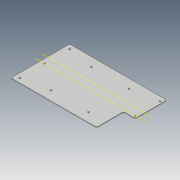
# Autodesk Inventor part: bottomMountingPlate
Saved by Autodesk Inventor 2018 (Build 220112000, 112)
## iProperties
Created: 2020-01-17
Part Number: bottomMountingPlate
Material: Generic
Document SubType Name: Modeling
Designer: anirudh.bali
Density: 1 g/cm^3
Appearance: Default
Author: anirudh.bali
Autodesk Inventor part; units mm, degrees
ref_plane "YZ Plane" through (0, 0, 0) normal (1, 0, 0) x (0, 1, 0)
ref_plane "XZ Plane" through (0, 0, 0) normal (0, 1, 0) x (-1, 0, 0)
ref_plane "XY Plane" through (0, 0, 0) normal (0, 0, 1) x (1, 0, 0)
sketch "Sketch1" plane through (0, 0, 0) normal (0, 1, 0) x (-1, 0, 0)
  line L0 (10.16, 0) -> (218.44, 0)
  line L1 (218.44, -165.1) -> (10.16, -165.1)
  circle A0 centre (218.44, -25.4) radius 1.75
  circle A1 centre (218.44, -82.55) radius 1.75
  circle A2 centre (218.44, -139.7) radius 1.75
  circle A3 centre (10.16, -25.4) radius 1.75
  circle A4 centre (10.16, -82.55) radius 1.75
  circle A5 centre (10.16, -139.7) radius 1.75
  line L2 (218.44, 0) -> (228.6, 0)
  line L3 (228.6, 0) -> (228.6, -165.1)
  line L4 (228.6, -165.1) -> (218.44, -165.1)
  line L5 (10.16, 0) -> (0, 0)
  line L6 (0, 0) -> (0, -165.1)
  line L7 (0, -165.1) -> (10.16, -165.1)
  dimension "d18" = 3.5
  dimension "d19" = 3.5
  dimension "d20" = 3.5
  dimension "d21" = 3.5
  dimension "d22" = 3.5
  dimension "d23" = 3.5
  dimension "d24" = 10.16
  constraints: 16 end point, 6 centre point, 3 horizontal, 2 collinear, 2 perpendicular, 1 parallel, 1 point on line
  measures "d18" diameter of A0
  measures "d19" diameter of A1
  measures "d20" diameter of A2
  measures "d21" diameter of A3
  measures "d22" diameter of A4
  measures "d23" diameter of A5
  measures "d24" distance of L0.end L2.end
extrude "Extrusion2" add sketch "Sketch1" along normal blind 1.5875
fillet "Fillet2" radius 3.175 4 edges at (0, 0.7937, 0) (0, 0.7937, -165.1) (-228.6, 0.7937, -165.1) (-228.6, 0.7937, 0)
sketch "Sketch2" plane through (0, 1.5875, 0) normal (0, 1, 0) x (1, 0, 0)
  line L0 (0, 161.925) -> (0, 3.175) projected
  line L1 (-228.6, 0) -> (0, 0)
  line L2 (0, 0) -> (0, 15.24)
  line L3 (0, 15.24) -> (-228.6, 15.24)
  line L4 (-228.6, 15.24) -> (-228.6, 0)
  line L5 (-228.6, 165.1) -> (0, 165.1)
  line L6 (0, 165.1) -> (0, 149.86)
  line L7 (0, 149.86) -> (-228.6, 149.86)
  line L8 (-228.6, 149.86) -> (-228.6, 165.1)
  dimension "d28" = 15.24
  dimension "d30" = 15.24
  constraints: 16 end point, 4 parallel, 2 horizontal, 2 perpendicular, 2 point on line
  measures "d28" distance of L2.end L1.end
  measures "d30" distance of L5.end L6.end
extrude "Extrusion3" cut sketch "Sketch2" against normal blind 1.5875
fillet "Fillet3" radius 3.175 4 edges at (-228.6, 0.7937, -15.24) (0, 0.7937, -15.24) (0, 0.7937, -149.86) (-228.6, 0.7937, -149.86)
ref_plane "Work Plane1" through (-3.175, 1.5875, -82.55) normal (0, 0, -1) x (-1, 0, 0)
ref_plane "Work Plane4" through (-3.175, 1.5875, -99.3521) normal (0, 0, -1) x (-1, 0, 0)
sketch "Sketch7" plane through (0, 1.5875, 0) normal (0, 1, 0) x (1, 0, 0)
  line L0 (0, 82.55) -> (-228.6, 82.55)
  line L1 (-228.6, 146.685) -> (-228.6, 18.415) projected
  line L2 (0, 82.55) -> (-228.6, 82.55)
  line L3 (-228.6, 18.415) -> (-228.6, 146.685) projected
  circle A0 centre (-70.953, 35.941) radius 1.75
  circle A1 centre (-70.953, 35.941) radius 1.75
  circle A2 centre (-157.647, 35.941) radius 1.75
  circle A3 centre (-157.647, 35.941) radius 1.75
  circle A4 centre (-157.647, 129.159) radius 1.75
  circle A5 centre (-70.953, 129.159) radius 1.75
  point P0 (0, 0)
  constraints: 6 centre point, 4 end point, 2 coincident, 1 midpoint, 1 perpendicular
extrude "Extrusion10" cut sketch "Sketch7" against normal blind 25.4
sketch "Sketch9" plane through (0, 1.5875, 0) normal (0, 1, 0) x (1, 0, 0)
  circle A0 centre (-10.16, 82.55) radius 1.75 projected
  circle A1 centre (-10.16, 82.55) radius 5.08
  line L0 (0, 15.24) -> (-31.75, 15.24)
  line L1 (-3.175, 15.24) -> (-225.425, 15.24) projected
  line L2 (-31.75, 15.24) -> (-31.75, 77.47)
  line L3 (-31.75, 77.47) -> (-10.16, 77.47)
  line L4 (-5.08, 82.55) -> (-5.08, 149.86)
  line L5 (-3.175, 149.86) -> (-225.425, 149.86) projected
  line L6 (-5.08, 149.86) -> (7.4371, 149.86)
  line L7 (7.4371, 149.86) -> (7.4371, 15.24)
  line L8 (7.4371, 15.24) -> (0, 15.24)
  point P0 (0, 0)
  dimension "d90" = 10.16
  dimension "d91" = 31.75
  constraints: 14 end point, 4 perpendicular, 2 point on circle, 2 point on line, 1 centre point, 1 coincident, 1 horizontal, 1 vertical
  measures "d90" diameter of A1
  measures "d91" distance of L0.start L0.end
extrude "Extrusion11" cut sketch "Sketch9" against normal blind 25.4 contours L4 L5 L6 L7 L8 L0 L2 L3 A1
fillet "Fillet5" radius 3.175 3 edges at (-31.75, 0.7937, -15.24) (-31.75, 0.7937, -77.47) (-5.08, 0.7937, -149.86)
sketch "Sketch10" plane through (0, 1.5875, 0) normal (0, 1, 0) x (1, 0, 0)
  circle A0 centre (-157.647, 35.941) radius 1.75 projected
  circle A1 centre (-157.647, 35.941) radius 1.75
  circle A2 centre (-70.953, 35.941) radius 1.75 projected
  circle A3 centre (-70.953, 35.941) radius 1.75
  circle A4 centre (-70.953, 129.159) radius 1.75 projected
  circle A5 centre (-70.953, 129.159) radius 1.75
  circle A6 centre (-157.647, 129.159) radius 1.75 projected
  circle A7 centre (-157.647, 129.159) radius 1.75
  line L0 (-157.647, 35.941) -> (-70.953, 35.941)
  line L1 (-70.953, 129.159) -> (-157.647, 129.159)
  point P0 (0, 0)
  constraints: 4 centre point, 4 coincident, 4 end point, 2 horizontal
body "Solid2"
